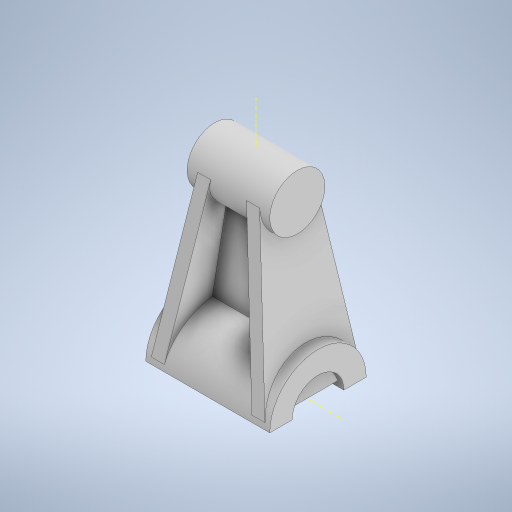
# Autodesk Inventor part: 05-15-2023 esercizi_piani parallaleli
Saved by Autodesk Inventor 2023 (Build 270158000, 158)
## iProperties
Created: 2023-05-15
Part Number: 05-15-2023 esercizi_piani parallaleli
Material: Generico
Document SubType Name: Modeling
Designer: Admin
Density: 1 g/cm^3
Appearance: Default
Author: Admin
Autodesk Inventor part; units mm, degrees
ref_plane "YZ Plane" through (0, 0, 0) normal (1, 0, 0) x (0, 1, 0)
ref_plane "XZ Plane" through (0, 0, 0) normal (0, 1, 0) x (-1, 0, 0)
ref_plane "XY Plane" through (0, 0, 0) normal (0, 0, 1) x (1, 0, 0)
sketch "Schizzo1" plane through (0, 0, 0) normal (1, 0, 0) x (0, 1, 0)
  circle A0 centre (96, 0) radius 10
  circle A1 centre (96, 0) radius 16
  arc A2 (0, -15) -> (0, 15) centre (0, 0) ccw
  arc A3 (0, -28) -> (0, 28) centre (0, 0) ccw
  line L0 (0, 28) -> (0, 15)
  line L1 (0, -15) -> (0, -28)
  line L2 (0, -8.9606) -> (0, 0)
  line L3 (0, 0) -> (192, 0)
  line L4 (3.5, 27.7804) -> (98, 15.8745)
  line L5 (98, -15.8745) -> (3.5, -27.7804)
  line L6 (0, 15) -> (0, -15)
  point P0 (9.0471, 0)
  point P1 (0, -4.4803)
  dimension "d0" = 20
  dimension "d1" = 15
  dimension "d2" = 96
  dimension "d3" = 28
  dimension "d4" = 32
  constraints: 14 end point, 8 point on circle, 5 coincident, 4 centre point, 4 tangent, 3 vertical, 2 midpoint, 2 vertical alignment, 1 collinear, 1 perpendicular
  measures "d0" diameter of A0
  measures "d1" radius of A2
  measures "d2" distance of A2.centre A0.centre
  measures "d3" radius of A3
  measures "d4" diameter of A1
extrude "Estrusione1" add sketch "Schizzo1" along normal mid plane 48 contours L3 A0 | L3 A1 A0 | A0 L3 A1 | A0 L3
extrude "Estrusione2" add sketch "Schizzo1" along normal mid plane 72 contours L3 A2 L0 A3 | A3 L1 A2 L3
sketch "Schizzo3" plane through (0, 0, 0) normal (1, 0, 0) x (0, 1, 0)
  line L0 (98, 15.8745) -> (3.5, 27.7804)
  circle A0 centre (96, 0) radius 16 projected
  arc A1 (0, -28) -> (0, 28) centre (0, 0) ccw projected
  constraints: 2 end point, 1 point on circle, 1 tangent, 3 other
ref_plane "Piano di lavoro2" through (0, 98, 15.8745) normal (0, 0.125, 0.9921567) x (-1, 0, 0)
sketch "Schizzo4" plane through (0, 98, 15.8745) normal (0, 0.125, 0.9921567) x (-1, 0, 0)
  line L0 (24, -16) -> (24, 16) projected
  line L1 (-24, 16) -> (-24, -16) projected
  line L2 (36, 67.247) -> (36, 98.747) projected
  line L3 (-36, 98.747) -> (-36, 67.247) projected
  line L4 (0, 95.247) -> (0, 93.372) construction
  line L5 (-18, 0) -> (-33, 95.247)
  line L6 (-10.4076, 0) -> (-25.4076, 95.247)
  line L7 (18, 0) -> (33, 95.247)
  line L8 (10.4076, 0) -> (25.4076, 95.247)
  line L9 (0, 0) -> (0, 95.247) projected
  line L10 (18, 0) -> (10.4076, 0)
  line L11 (-10.4076, 0) -> (-18, 0)
  line L12 (-25.4076, 95.247) -> (-33, 95.247)
  line L13 (36, 93.372) -> (-36, 93.372) projected
  line L14 (33, 95.247) -> (25.4076, 95.247)
  line L15 (36, 97.122) -> (-36, 97.122) projected
  point P0 (36, 91.747)
  point P1 (-36, 91.747)
  dimension "d10" = 7.5
  dimension "d11" = 36
  dimension "d12" = 66
  constraints: 18 end point, 4 horizontal alignment, 4 symmetric about line, 3 parallel, 1 collinear, 1 horizontal, 1 midpoint, 1 vertical
  measures "d10" distance between parallel lines of L5 L6
  measures "d11" distance of L5.start L7.start
  measures "d12" distance of L5.end L7.end
sketch "Schizzo6" plane through (0, 0, 0) normal (0, 0, 1) x (1, 0, 0)
  line L0 (-18, 98) -> (-33, 3.5) projected
  line L1 (-10.4076, 98) -> (-25.4076, 3.5) projected
  line L2 (10.4076, 98) -> (25.4076, 3.5) projected
  line L3 (18, 98) -> (33, 3.5) projected
  line L4 (-36, 0) -> (36, 0) projected
  line L5 (36, 0) -> (36, 0) projected
  line L6 (36, 0) -> (-36, 0) projected
  line L7 (-36, 0) -> (-36, 0) projected
  line L8 (-33, 3.5) -> (-25.4076, 3.5) projected
  line L9 (25.4076, 3.5) -> (33, 3.5) projected
  line L10 (-18, 98) -> (-10.4076, 98) projected
  line L11 (10.4076, 98) -> (18, 98) projected
  point P0 (0, 0)
extrude "Estrusione4" add sketch "Schizzo6" along normal up to surface surface through (0, 98, 15.8745) normal (0, 0.125, 0.9921567)
mirror "Specchio1" about plane through (0, 0, 0) normal (0, 0, 1) of "Estrusione4"
sketch "Schizzo8" plane through (0, 0, 0) normal (1, 0, 0) x (0, 1, 0)
  circle A0 centre (96, 0) radius 16 projected
  arc A1 (0, -28) -> (0, 28) centre (0, 0) ccw projected
  line L0 (80.4457, 3.75) -> (27.7477, 3.75)
  line L1 (80.4457, -3.75) -> (27.7477, -3.75)
  line L2 (-22.7749, 0) -> (136.6494, 0) construction
  dimension "d17" = 7.5
  constraints: 4 end point, 4 point on circle, 1 horizontal, 1 parallel, 1 other
  measures "d17" distance between parallel lines of L1 L0
extrude "Estrusione5" add sketch "Schizzo8" along normal up to surface contours A0 L1 A1 L0 surface through (10.4076, 98, 0) normal (-0.9876355, -0.1567675, 0)
extrude "Estrusione6" add sketch "Schizzo8" against normal up to surface contours A0 L1 A1 L0 surface through (-25.4076, 3.5, 0) normal (0.9876355, -0.1567675, 0)
sketch "Schizzo9" plane through (0, 0, 0) normal (0, 0, 1) x (1, 0, 0)
  line L0 (-50.4, 0) -> (50.4, 0) projected
  line L1 (0, -22.7749) -> (0, 136.6494) projected
  point P0 (0, 0)
